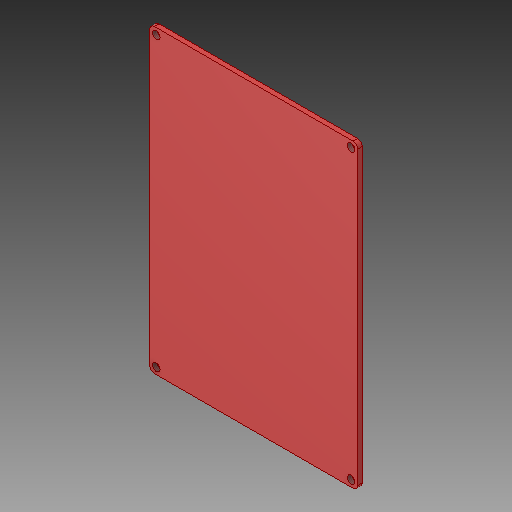
# Autodesk Inventor part: Door Plate
Saved by Autodesk Inventor 2018 (Build 220112000, 112)
## iProperties
Created: 2018-02-10
Part Number: Door Plate
Material: PC/ABS Plastic
Document SubType Name: Modeling
Designer: Joey
Density: 0.357273 g/cm^3
Appearance: Smooth - Red
Author: Joey
Autodesk Inventor part; units mm, degrees
ref_plane "YZ Plane" through (0, 0, 0) normal (1, 0, 0) x (0, 1, 0)
ref_plane "XZ Plane" through (0, 0, 0) normal (0, 1, 0) x (-1, 0, 0)
ref_plane "XY Plane" through (0, 0, 0) normal (0, 0, 1) x (1, 0, 0)
sketch "Sketch1" plane through (0, 0, 0) normal (0, 0, 1) x (1, 0, 0)
  circle A0 centre (101.9076, -14.556) radius 5.2959 construction
  line L0 (89.2076, -40.4217) -> (89.2076, -1.856) construction
  line L1 (89.2076, -40.4217) -> (127.7733, -1.856) construction
  line L2 (89.2076, -1.856) -> (127.7733, -1.856) construction
  circle A1 centre (369.0061, -14.556) radius 5.2959 construction
  line L3 (381.7061, -1.856) -> (381.7061, -40.4217) construction
  line L4 (343.1404, -1.856) -> (381.7061, -1.856) construction
  line L5 (343.1404, -1.856) -> (381.7061, -40.4217) construction
  circle A2 centre (369.0061, -408.7889) radius 5.2959 construction
  line L6 (381.7061, -382.9233) -> (381.7061, -421.4889) construction
  line L7 (381.7061, -382.9233) -> (343.1404, -421.4889) construction
  line L8 (381.7061, -421.4889) -> (343.1404, -421.4889) construction
  circle A3 centre (101.9076, -408.7889) radius 5.2959 construction
  line L9 (89.2076, -421.4889) -> (89.2076, -382.9233) construction
  line L10 (127.7733, -421.4889) -> (89.2076, -421.4889) construction
  line L11 (127.7733, -421.4889) -> (89.2076, -382.9233) construction
  line L12 (377.8961, -417.6789) -> (93.0176, -417.6789)
  line L13 (93.0176, -417.6789) -> (93.0176, -5.666)
  line L14 (93.0176, -5.666) -> (377.8961, -5.666)
  line L15 (377.8961, -5.666) -> (377.8961, -417.6789)
  point P0 (0, 0)
  dimension "d0" = 3.81
  dimension "d1" = 3.81
  dimension "d2" = 3.81
  dimension "d3" = 3.81
  constraints: 8 end point, 2 parallel, 1 horizontal, 1 perpendicular
  measures "d0" distance between parallel lines of L14 L2
  measures "d1" distance between parallel lines of L13 L0
  measures "d2" distance between parallel lines of L15 L3
  measures "d3" distance between parallel lines of L10 L12
extrude "Extrusion1" add sketch "Sketch1" along normal blind 6.35
sketch "Sketch2" plane through (0, 0, 6.35) normal (0, 0, 1) x (1, 0, 0)
  circle A0 centre (101.9076, -14.556) radius 5.2959 construction
  line L0 (89.2076, -40.4217) -> (89.2076, -1.856) construction
  line L1 (89.2076, -40.4217) -> (127.7733, -1.856) construction
  line L2 (89.2076, -1.856) -> (127.7733, -1.856) construction
  circle A1 centre (369.0061, -14.556) radius 5.2959 construction
  line L3 (381.7061, -1.856) -> (381.7061, -40.4217) construction
  line L4 (343.1404, -1.856) -> (381.7061, -1.856) construction
  line L5 (343.1404, -1.856) -> (381.7061, -40.4217) construction
  circle A2 centre (369.0061, -408.7889) radius 5.2959 construction
  line L6 (381.7061, -382.9233) -> (381.7061, -421.4889) construction
  line L7 (381.7061, -382.9233) -> (343.1404, -421.4889) construction
  line L8 (381.7061, -421.4889) -> (343.1404, -421.4889) construction
  circle A3 centre (101.9076, -408.7889) radius 5.2959 construction
  line L9 (89.2076, -421.4889) -> (89.2076, -382.9233) construction
  line L10 (127.7733, -421.4889) -> (89.2076, -421.4889) construction
  line L11 (127.7733, -421.4889) -> (89.2076, -382.9233) construction
  point P0 (0, 0)
  constraints: 4 coincident
hole "Hole1" at (101.9076, -14.556, 6.35) at (369.0061, -14.556, 6.35) at (369.0061, -408.7889, 6.35) at (101.9076, -408.7889, 6.35) direction (0, 0, -1) diameter 10.5918 end through all thread size "1/2-13 UNC" class "2B" standard "ANSI Unified Screw Threads"
fillet "Fillet1" radius 6.35 4 edges at (93.0176, -5.666, 3.175) (377.8961, -5.666, 3.175) (377.8961, -417.6789, 3.175) (93.0176, -417.6789, 3.175)
body "Solid1"
